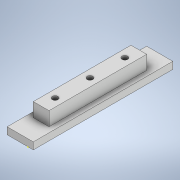
# Autodesk Inventor part: Pin holder
Saved by Autodesk Inventor 2022 (Build 260153000, 153)
## iProperties
Created: 2022-02-25
Part Number: Pin holder
Material: Generic
Document SubType Name: Modeling
Designer: Alexa
Density: 1 g/cm^3
Appearance: Default
Author: Alexa
Autodesk Inventor part; units mm, degrees
ref_plane "YZ Plane" through (0, 0, 0) normal (1, 0, 0) x (0, 1, 0)
ref_plane "XZ Plane" through (0, 0, 0) normal (0, 1, 0) x (-1, 0, 0)
ref_plane "XY Plane" through (0, 0, 0) normal (0, 0, 1) x (1, 0, 0)
sketch "Sketch1" plane through (0, 0, 0) normal (0, 1, 0) x (-1, 0, 0)
  line L0 (0, 0) -> (15, 0)
  line L1 (15, 0) -> (15, -80)
  line L2 (15, -80) -> (0, -80)
  line L3 (0, -80) -> (0, 0)
  dimension "d0" = 15
  dimension "d1" = 80
  constraints: 8 end point, 2 parallel, 1 horizontal, 1 perpendicular
  measures "d0" distance of L1.end L2.end
  measures "d1" distance of L0.end L1.end
extrude "Extrusion1" add sketch "Sketch1" along normal blind 4
sketch "Sketch2" plane through (0, 4, 0) normal (0, 1, 0) x (1, 0, 0)
  line L0 (-15, 80) -> (-15, 0) projected
  line L1 (0, 0) -> (0, 80) projected
  line L2 (-15, 80) -> (0, 80)
  line L3 (0, 80) -> (0, 0)
  line L4 (0, 0) -> (-15, 0)
  line L5 (-15, 0) -> (-15, 80)
  line L6 (-15, 0) -> (0, 0) projected
  line L7 (-15, 80) -> (-7.5, 80)
  line L8 (-7.5, 80) -> (-7.5, 0)
  line L9 (-7.5, 0) -> (-15, 0)
  line L10 (-15, 0) -> (-15, 80)
  line L11 (-7.5, 0) -> (-7.5, 20)
  line L12 (-7.5, 20) -> (-7.5, 40)
  line L13 (-7.5, 40) -> (-7.5, 60)
  circle A0 centre (-7.5, 60) radius 1.65
  circle A1 centre (-7.5, 40) radius 1.65
  circle A2 centre (-7.5, 20) radius 1.65
  line L14 (-7.5, 80) -> (-7.5, 68)
  line L15 (-7.5, 0) -> (-7.5, 12)
  line L16 (-12, 68) -> (-3, 68)
  line L17 (-3, 68) -> (-3, 12)
  line L18 (-3, 12) -> (-12, 12)
  line L19 (-12, 12) -> (-12, 68)
  dimension "d4" = 20
  dimension "d5" = 20
  dimension "d6" = 20
  dimension "d7" = 3.3
  dimension "d8" = 3.3
  dimension "d9" = 3.3
  dimension "d10" = 12
  dimension "d11" = 12
  dimension "d12" = 9
  constraints: 34 end point, 6 parallel, 4 point on line, 3 centre point, 3 coincident, 3 horizontal, 3 perpendicular, 2 midpoint
  measures "d4" distance of L8.end L11.end
  measures "d5" distance of L11.end L12.end
  measures "d6" distance of L12.end L13.end
  measures "d7" diameter of A0
  measures "d8" diameter of A1
  measures "d9" diameter of A2
  measures "d10" distance of L7.end L14.end
  measures "d11" distance of L8.end L15.end
  measures "d12" distance of L17.end L18.end
extrude "Extrusion2" add sketch "Sketch2" along normal blind 8 contours L16 L17 L18 L8 A2 A1 A0 | L8 A0 A1 A2 L18 L19 L16
sketch "Sketch3" plane through (-3, 4, -12) normal (1, 0, 0) x (0, 0, -1)
  point P0 (-12, -4)
body "Solid1"
